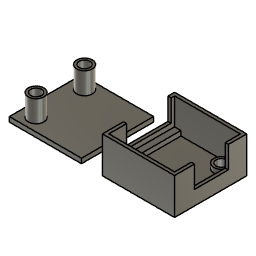
Endstop Case v1 (Autodesk Fusion 360 design; units mm, degrees)
Autodesk Fusion 360 part; units mm, degrees
note: some values were not read from the file. Set by a fixed rule: which face or edge a step refers to.
sketch "Skizze4" plane through (0, 0, 0) normal (0, 0, 1) x (1, 0, 0)
  line L0 (10.325, -10.325) -> (-10.325, -10.325)
  line L1 (-10.325, -10.325) -> (-10.325, 10.325)
  line L2 (-10.325, 10.325) -> (10.325, 10.325)
  line L3 (10.325, 10.325) -> (10.325, -10.325)
  line L4 (10.325, -10.325) -> (-10.325, 10.325) construction
  line L5 (-10.325, -10.325) -> (10.325, 10.325) construction
  line L6 (11.325, -11.325) -> (-11.325, -11.325)
  line L7 (-11.325, -11.325) -> (-11.325, 11.325)
  line L8 (-11.325, 11.325) -> (11.325, 11.325)
  line L9 (11.325, 11.325) -> (11.325, -11.325)
  dimension "d10" = 20.65
  dimension "d11" = 20.65
  dimension "d14" = -1
  constraint horizontal L0
  constraint perpendicular L0 L1
  constraint parallel L0 L2
  constraint parallel L1 L3
  constraint coincident L4 origin
  constraint coincident L5 origin
  measures "d10" distance of L1.end L2.end
  measures "d11" distance of L0.end L1.end
extrude "Extrusion4" add sketch "Skizze4" along normal blind 1.5 contours L0 L1 L2 L3 makes body 1
extrude "Extrusion5" add sketch "Skizze4" along normal blind 11.4 bodies 1
sketch "Skizze5" plane through (0, 0, 1.5) normal (0, 0, 1) x (-1, 0, 0)
  line L0 (-10.325, -10.325) -> (10.325, -10.325)
  line L1 (10.325, -10.325) -> (10.325, 10.325)
  line L2 (10.325, 10.325) -> (-10.325, 10.325)
  line L3 (-10.325, 10.325) -> (-10.325, -10.325)
hole "Bohrung1" at (6.875, 7.875, 1.5) direction (0, 0, -1) diameter 3.4 depth 8 tip angle 118 bodies 1
hole "Bohrung2" at (6.875, -7.375, 1.5) direction (0, 0, -1) diameter 3.4 depth 8 tip angle 118 bodies 1
sketch "Skizze6" plane through (0, 0, 1.5) normal (0, 0, 1) x (-1, 0, 0)
  circle A0 centre (-6.875, 7.375) radius 1.7
  circle A1 centre (-6.875, -7.875) radius 1.7
  line L0 (-10.325, -10.325) -> (10.325, -10.325)
  line L1 (10.325, -10.325) -> (10.325, 10.325)
  line L2 (10.325, 10.325) -> (-10.325, 10.325)
  line L3 (-10.325, 10.325) -> (-10.325, -10.325)
  circle A2 centre (-6.875, -7.875) radius 1.7
  circle A3 centre (-6.875, -7.875) radius 2.45
  circle A4 centre (-6.875, 7.375) radius 1.7
  circle A5 centre (-6.875, 7.375) radius 2.45
  line L4 (10.325, -10.325) -> (8.325, -10.325)
  line L5 (8.325, -10.325) -> (8.325, 10.325)
  line L6 (8.325, 10.325) -> (10.325, 10.325)
  line L7 (10.325, 10.325) -> (10.325, -10.325)
  dimension "d27" = 0.75
  dimension "d28" = 0.75
  dimension "d31" = 2
  constraint concentric A1 A2
  constraint concentric A0 A4
  constraint horizontal L4
  constraint vertical L5
  constraint horizontal L6
  constraint vertical L7
  constraint coincident L2 L5.end
  constraint coincident L0.end L1.start
  measures "d31" distance of L0.end L4.end
extrude "Extrusion6" add sketch "Skizze6" along normal blind 1.5 separate body contours A3 | A5 makes body 2 at (4.4372, 8.1189, 2) makes body 3 at (4.428, -7.2529, 2.5)
extrude "Extrusion7" add sketch "Skizze6" along normal blind 1.5 contours L0 L1 L2 L4 L5 L6 L7 bodies 1
sketch "Skizze7" plane through (-10.325, 0, 0) normal (1, 0, 0) x (0, 1, 0)
  line L0 (-10.325, 3) -> (10.325, 3)
  line L1 (10.325, 3) -> (10.325, 11.4)
  line L2 (10.325, 11.4) -> (-10.325, 11.4)
  line L3 (-10.325, 11.4) -> (-10.325, 3)
  line L4 (9.25, 11.4) -> (-4.75, 11.4)
  line L5 (-4.75, 11.4) -> (-4.75, 4.5)
  line L6 (-4.75, 4.5) -> (9.25, 4.5)
  line L7 (9.25, 4.5) -> (9.25, 11.4)
  constraint horizontal L4
  constraint vertical L5
  constraint horizontal L6
  constraint vertical L7
  constraint coincident L2 L4.start
sketch "Skizze8" plane through (11.325, 0, 0) normal (1, 0, 0) x (0, 1, 0)
  line L0 (-11.325, 0) -> (11.325, 0)
  line L1 (11.325, 0) -> (11.325, 11.4)
  line L2 (11.325, 11.4) -> (-11.325, 11.4)
  line L3 (-11.325, 11.4) -> (-11.325, 0)
  line L4 (-5.1, 11.4) -> (5.6, 11.4)
  line L5 (5.6, 11.4) -> (5.6, 4.5)
  line L6 (5.6, 4.5) -> (-5.1, 4.5)
  line L7 (-5.1, 4.5) -> (-5.1, 11.4)
  constraint horizontal L4
  constraint vertical L5
  constraint horizontal L6
  constraint vertical L7
  constraint coincident L2 L4.start
extrude "Extrusion8" cut sketch "Skizze8" against normal blind 1.5 contours L2 L4 L5 L6 L7 bodies 1
extrude "Extrusion9" cut sketch "Skizze7" against normal blind 1.5 contours L2 L4 L5 L6 L7 bodies 1
sketch "Skizze9" plane through (0, 0, 11.4) normal (0, 0, 1) x (-1, 0, 0)
  line L0 (11.325, -9.25) -> (10.325, -9.25)
  line L1 (10.325, -9.25) -> (10.325, -10.325)
  line L2 (10.325, -10.325) -> (-10.325, -10.325)
  line L3 (-10.325, -10.325) -> (-10.325, -5.6)
  line L4 (-10.325, -5.6) -> (-11.325, -5.6)
  line L5 (-11.325, -5.6) -> (-11.325, -11.325)
  line L6 (-11.325, -11.325) -> (11.325, -11.325)
  line L7 (11.325, -11.325) -> (11.325, -9.25)
  line L8 (11.325, -11.325) -> (-11.275, -11.325)
  line L9 (-11.275, -11.325) -> (-11.275, 11.275)
  line L10 (-11.275, 11.275) -> (11.325, 11.275)
  line L11 (11.325, 11.275) -> (11.325, -11.325)
  dimension "d38" = 22.6
  dimension "d39" = 22.6
  constraint horizontal L8
  constraint vertical L9
  constraint horizontal L10
  constraint vertical L11
  constraint coincident L6.end L7.start
  measures "d38" distance of L6.end L8.end
  measures "d39" distance of L6.end L10.end
extrude "Extrusion10" add sketch "Skizze9" along normal blind 1.5 separate body contours L0 L1 L2 L3 L4 L6 L7 L8 L9 L11 | L0 L1 L2 L3 L4 L9 L10 L11 makes body 4
move_face "Flächen versetzen1" offset 0.05 1 faces at (3.7417, -11.275, 11.9) on bodies 4
move_face "Flächen versetzen2" offset 0.05 2 faces at (11.275, 9.4167, 11.9) (11.275, -0.0417, 11.9) on bodies 4
hole "Bohrung3" at (6.888, 7.857, 12.9) direction (0, 0, -1) diameter 3.4 depth 8 tip angle 118 bodies 4
hole "Bohrung4" at (6.889, -7.364, 12.9) direction (0, 0, -1) diameter 3.4 depth 8 tip angle 118 bodies 4
sketch "Skizze10" plane through (0, 0, 11.4) normal (0, 0, -1) x (1, 0, 0)
  circle A0 centre (6.889, 7.364) radius 1.7
  circle A1 centre (6.888, -7.857) radius 1.7
  line L0 (11.325, 11.325) -> (-11.325, 11.325)
  line L1 (-11.325, 11.325) -> (-11.325, -11.325)
  line L2 (-11.325, -11.325) -> (11.325, -11.325)
  line L3 (11.325, -11.325) -> (11.325, 11.325)
  circle A2 centre (6.889, 7.364) radius 1.7
  circle A3 centre (6.889, 7.364) radius 2.45
  circle A4 centre (6.888, -7.857) radius 1.7
  circle A5 centre (6.888, -7.857) radius 2.45
  dimension "d52" = 0.75
  dimension "d53" = 0.75
  constraint concentric A0 A2
  constraint concentric A1 A4
extrude "Extrusion11" add sketch "Skizze10" along normal blind 6.8 contours A3 | A5 bodies 4
move_body "Verschieben4" bodies 4 to x (-1, 0, 0) y (0, 1, 0) z (0, 0, -1) at (-29.2313, 0, 12.9)
combine "Kombinieren1" operation add target body 1 tool bodies 2 3
move_face "Fläche verschieben1" by (61, 0, 0) 1 faces at (-23.2418, -2.1003, 1.5) on bodies 4
named bodies: "Base", "Deckel"
